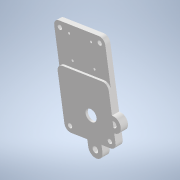
# Autodesk Inventor part: Пластина 1
Saved by Autodesk Inventor 2021 (Build 250183000, 183)
## iProperties
Created: 2020-12-07
Part Number: Пластина 1
Material: Типовые
Document SubType Name: Modeling
Designer: User
Density: 1 g/cm^3
Appearance: По умолчанию
Author: User
Autodesk Inventor part; units mm, degrees
sketch "Эскиз1" plane through (0, 0, 0) normal (0, 0, 1) x (1, 0, 0)
  circle A0 centre (0, 0) radius 14 projected
  circle A1 centre (-4.693, 29.6307) radius 12 projected
  line L0 (20.6222, 100.5641) -> (40.3486, -23.9834)
  line L1 (40.3486, -23.9834) -> (-30.9625, -35.2779)
  line L2 (-30.9625, -35.2779) -> (-50.6889, 89.2696)
  line L3 (-50.6889, 89.2696) -> (20.6222, 100.5641)
  line L4 (7.1366, 89.8223) -> (12.6431, 55.0556) construction
  line L5 (-31.6345, 87.2252) -> (3.1321, 92.7317) construction
  line L6 (-29.0374, 48.4541) -> (-34.5439, 83.2207) construction
  point P0 (0, 0)
  dimension "d0" = 15
  dimension "d1" = 15
  dimension "d2" = 5
  dimension "d3" = 30
  constraints: 8 end point, 4 parallel, 1 perpendicular
  measures "d0" distance between parallel lines of L0 L4
  measures "d1" distance between parallel lines of L2 L6
  measures "d2" distance between parallel lines of L3 L5
  measures "d3" distance from line of L1 A0.centre
ref_plane "РабПлоскость1" through (-35.2416, 44.847, 7) normal (0, 0, -1) x (-0.1564345, 0.9876883, 0)
extrude "Выдавливание1" add sketch "Эскиз1" along normal up to surface (7 mm away)
sketch "Эскиз2" plane through (40.3486, -23.9834, 7) normal (0, 0, 1) x (0.9876883, 0.1564345, 0)
  circle A0 centre (-36.1, 60) radius 12 projected
  point P0 (-36.1, 30)
ref_plane "РабПлоскость2" through (-17.9323, 16.3914, 6) normal (0, 0, 1) x (0.9876885, 0.1564338, 0)
extrude "Выдавливание2" add sketch "Эскиз2" against normal up to surface (1 mm away)
sketch "Эскиз3" plane through (40.3486, -23.9834, 7) normal (0, 0, 1) x (0.9876883, 0.1564345, 0)
  line L0 (-72.2, 126.1) -> (-72.2, 0) projected
  line L1 (0, 0) -> (0, 126.1) projected
  line L2 (-72.2, 0) -> (0, 0)
  line L3 (0, 0) -> (0, 75.9)
  line L4 (0, 75.9) -> (-72.2, 75.9)
  line L5 (-72.2, 75.9) -> (-72.2, 0)
  line L6 (-18.5, 78.9) -> (-53.7, 78.9) construction
  circle A0 centre (-36.1, 30) radius 7.5
  point P0 (0, 0)
  point P1 (-72.2, 75.9)
  dimension "d8" = 3
  dimension "d34" = 15
  constraints: 8 end point, 2 parallel, 1 centre point, 1 coincident, 1 horizontal, 1 perpendicular, 1 point on line
  measures "d8" distance between parallel lines of L6 L4
  measures "d34" diameter of A0
ref_plane "РабПлоскость3" through (-9.421, -9.421, 10) normal (0, 0, 1) x (1, 0, 0)
extrude "Выдавливание3" add sketch "Эскиз3" along normal up to surface (3 mm away)
fillet "Сопряжение1" radius 0.5 1 edges at (-7.4077, -1.1733, 10)
fillet "Сопряжение2" radius 8 6 edges at (-50.6889, 89.2696, 3.5) (-30.9625, -35.2779, 5) (40.3486, -23.9834, 5) (20.6222, 100.5641, 3.5) (28.4752, 50.9822, 8.5) (-42.8359, 39.6876, 8.5)
sketch "Эскиз4" plane through (0, 0, 0) normal (0, 0, -1) x (-1, 0, 0)
  arc A0 (-12.7207, 99.3127) -> (-21.8737, 92.6626) centre (-13.9722, 91.4112) ccw construction
  arc A1 (49.4374, 81.3681) -> (42.7874, 90.521) centre (41.5359, 82.6195) ccw construction
  arc A2 (23.061, -34.0265) -> (32.214, -27.3764) centre (24.3125, -26.125) ccw construction
  arc A3 (-39.0971, -16.0819) -> (-32.4471, -25.2348) centre (-31.1956, -17.3333) ccw construction
  point P0 (0, 0)
hole "Отверстие1" at (31.1956, -17.3333, 0) at (-24.3125, -26.125, 0) at (-41.5359, 82.6195, 0) at (13.9722, 91.4112, 0) direction (0, 0, 1) diameter 6 end through all clearance for "с потайной головкой ГОСТ 12876-67" size "M6" standard "ГОСТ"
sketch "Эскиз5" plane through (0, 0, 0) normal (0, 0, -1) x (-1, 0, 0)
  circle A0 centre (23.8348, 51.4043) radius 1.5 construction
  circle A1 centre (-6.7835, 56.2537) radius 1.5 construction
  circle A2 centre (-1.934, 86.8721) radius 1.5 construction
  circle A3 centre (28.6843, 82.0226) radius 1.5 construction
  point P0 (0, 0)
hole "Отверстие2" at (-23.8348, 51.4043, 0) at (-28.6843, 82.0226, 0) at (1.934, 86.8721, 0) at (6.7835, 56.2537, 0) direction (0, 0, 1) diameter 3 end through all countersink diameter 6.6 countersink angle 90 clearance for "с потайной головкой ГОСТ 12876-67" size "M3" standard "ГОСТ"
sketch "Эскиз6" plane through (0, 0, 0) normal (0, 0, -1) x (-1, 0, 0)
  line L0 (-31.1854, 39.6237) -> (-41.9794, -28.5268) construction
  line L1 (-38.6544, -33.1033) -> (16.6561, -41.8636) construction
  circle A0 centre (-36.5824, 5.5484) radius 4
  circle A1 centre (-10.9991, -37.4835) radius 4
  arc A2 (-35.0181, 15.4253) -> (-38.1468, -4.3285) centre (-36.5824, 5.5484) ccw
  line L2 (-38.1468, -4.3285) -> (-32.3194, -5.2514)
  line L3 (-35.0181, 15.4253) -> (-29.1907, 14.5023)
  arc A3 (-20.876, -35.9191) -> (-1.1222, -39.0478) centre (-10.9991, -37.4835) ccw
  line L4 (-20.876, -35.9191) -> (-19.5084, -27.2841)
  line L5 (-1.1222, -39.0478) -> (0.2454, -30.4128)
  line L6 (-27.5086, -26.017) -> (18.1226, -33.2443)
  line L7 (-39.0971, -16.0819) -> (-21.8737, 92.6626) projected
  point P0 (0, 0)
  point P1 (-38.1468, -4.3285)
  point P2 (-21.8737, 92.6626)
  point P3 (-37.2579, -4.4693)
  point P4 (-34.1292, 15.2845)
  dimension "d27" = 8
  dimension "d28" = 8
  dimension "d29" = 10
  dimension "d30" = 10
  dimension "d31" = 10
  constraints: 10 end point, 4 centre point, 4 point on circle, 4 point on line, 2 coincident, 2 midpoint, 2 perpendicular, 1 parallel, 3 other
  measures "d27" diameter of A0
  measures "d28" diameter of A1
  measures "d29" radius of A2
  measures "d30" distance from line of A0.centre L2
  measures "d31" radius of A3
extrude "Выдавливание4" add sketch "Эскиз6" against normal up to surface (10 mm away) contours A0 L7 L2 A2 L3 | L4 L6 L5 A3
sketch "Эскиз7" plane through (-32.214, -27.3764, 10) normal (0, 0, 1) x (0.9876883, 0.1564345, 0)
  arc A0 (72.2, 17.8599) -> (72.2, 25.6548) centre (73.1, 21.7574) ccw projected
  circle A1 centre (73.1, 21.7574) radius 4
  point P0 (36.1, 22)
  constraints: 1 centre point, 1 coincident, 1 concentric
extrude "Выдавливание5" cut sketch "Эскиз7" against normal through all
equation "\"d1\" = d0"
equation "\"d28\" = d27"
equation "\"d30\" = d29"
equation "\"d31\" = d29"
